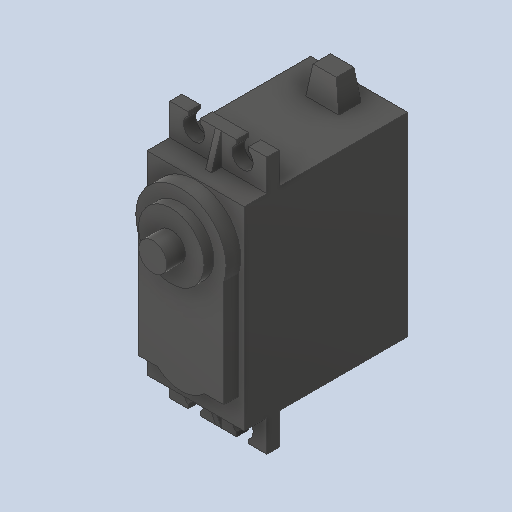
# Autodesk Inventor part: servo motor HS-7955TG
Saved by Autodesk Inventor 2022 (Build 260153000, 153)
## iProperties
Created: 2017-12-19
Part Number: servo motor HS-7955TG
Material: Generic
Document SubType Name: Modeling
Designer: s41607
Density: 1 g/cm^3
Appearance: Smooth - Dark Gray
Author: s41607
Autodesk Inventor part; units mm, degrees
ref_plane "YZ Plane" through (0, 0, 0) normal (1, 0, 0) x (0, 1, 0)
ref_plane "XZ Plane" through (0, 0, 0) normal (0, 1, 0) x (-1, 0, 0)
ref_plane "XY Plane" through (0, 0, 0) normal (0, 0, 1) x (1, 0, 0)
sketch "Sketch1" plane through (0, 0, 0) normal (0, 0, 1) x (1, 0, 0)
  line L0 (-14, 0) -> (14, 0) projected
  line L1 (0, 28) -> (0, -28) projected
  line L2 (-10, 20) -> (10, 20)
  line L3 (10, 20) -> (10, -20)
  line L4 (10, -20) -> (-10, -20)
  line L5 (-10, -20) -> (-10, 20)
  point P0 (0, 0)
  dimension "d0" = 20
  dimension "d1" = 40
  constraints: 8 end point, 2 parallel, 1 horizontal, 1 perpendicular, 2 other
  measures "d0" distance of L2.start L2.end
  measures "d1" distance of L4.end L2.start
extrude "Extrusion1" add sketch "Sketch1" along normal blind 7.2 and the other way blind 26.5
sketch "Sketch2" plane through (0, 0, 0) normal (0, 0, 1) x (1, 0, 0)
  line L0 (-14, 0) -> (14, 0) projected
  line L1 (0, 28) -> (0, -28) projected
  line L2 (-10, 20) -> (-10, -20) projected
  line L3 (10, -20) -> (10, 20) projected
  line L4 (-10, 26.5) -> (10, 26.5)
  line L5 (10, 26.5) -> (10, -26.5)
  line L6 (10, -26.5) -> (-10, -26.5)
  line L7 (-10, -26.5) -> (-10, 26.5)
  point P0 (0, 0)
  dimension "d6" = 53
  constraints: 8 end point, 2 collinear, 2 parallel, 1 horizontal, 1 perpendicular, 1 other
  measures "d6" distance of L6.end L4.start
extrude "Extrusion2" add sketch "Sketch2" along normal blind 2.5
sketch "Sketch3" plane through (0, 0, 0) normal (0, 0, 1) x (1, 0, 0)
  line L0 (0, 37.1) -> (0, -37.1) projected
  line L1 (-14, 0) -> (14, 0) projected
  line L2 (-5, 23.925) -> (5, 23.925) construction
  line L3 (5, 23.925) -> (5, -23.925) construction
  line L4 (5, -23.925) -> (-5, -23.925) construction
  line L5 (-5, -23.925) -> (-5, 23.925) construction
  point P0 (0, 0)
  dimension "d9" = 47.85
  dimension "d10" = 10
  constraints: 8 end point, 4 coincident, 2 parallel, 1 horizontal, 1 perpendicular, 2 other
  measures "d9" distance of L2.end L3.end
  measures "d10" distance of L2.start L2.end
hole "Hole1" at (5, 23.925, 0) at (-5, 23.925, 0) at (-5, -23.925, 0) at (5, -23.925, 0) direction (0, 0, 1) diameter 4.35 depth 8 tip angle 118
sketch "Sketch4" plane through (0, 0, 0) normal (0, 0, 1) x (1, 0, 0)
  line L0 (-14, 0) -> (14, 0) projected
  line L1 (0, 37.1) -> (0, -37.1) projected
  line L2 (10, 26.5) -> (-10, 26.5) projected
  line L3 (-10, -26.5) -> (10, -26.5) projected
  circle A0 centre (-5, 23.925) radius 2.175 projected
  circle A1 centre (5, 23.925) radius 2.175 projected
  circle A2 centre (-5, -23.925) radius 2.175 projected
  circle A3 centre (5, -23.925) radius 2.175 projected
  line L4 (-6.25, -23.925) -> (-3.75, -23.925)
  line L5 (-3.75, -23.925) -> (-3.75, -26.5)
  line L6 (-3.75, -26.5) -> (-6.25, -26.5)
  line L7 (-6.25, -26.5) -> (-6.25, -23.925)
  line L8 (6.25, -23.925) -> (3.75, -23.925)
  line L9 (3.75, -23.925) -> (3.75, -26.5)
  line L10 (3.75, -26.5) -> (6.25, -26.5)
  line L11 (6.25, -26.5) -> (6.25, -23.925)
  line L12 (-10, 26.5) -> (10, 26.5) projected
  line L13 (6.25, 26.5) -> (3.75, 26.5)
  line L14 (3.75, 26.5) -> (3.75, 23.925)
  line L15 (3.75, 23.925) -> (6.25, 23.925)
  line L16 (6.25, 23.925) -> (6.25, 26.5)
  line L17 (-3.75, 26.5) -> (-6.25, 26.5)
  line L18 (-6.25, 26.5) -> (-6.25, 23.925)
  line L19 (-6.25, 23.925) -> (-3.75, 23.925)
  line L20 (-3.75, 23.925) -> (-3.75, 26.5)
  point P0 (0, 0)
  dimension "d18" = 2.5
  dimension "d19" = 2.5
  dimension "d20" = 2.5
  dimension "d21" = 2.5
  constraints: 32 end point, 8 parallel, 4 coincident, 4 horizontal, 4 midpoint, 4 perpendicular, 4 point on line
  measures "d18" distance between parallel lines of L7 L5
  measures "d19" distance between parallel lines of L11 L9
  measures "d20" distance between parallel lines of L16 L14
  measures "d21" distance between parallel lines of L20 L18
extrude "Extrusion3" cut sketch "Sketch4" along normal through all contours L9 A3 L11 L3 | L3 L7 A2 L5 | L2 L16 A1 L14 | L20 A0 L18 L2 | A1 L16 L15 L14 | L20 L19 L18 A0 | A2 L7 L4 L5 | L9 L8 L11 A3 picked at (4.9114, 24.6446) picked at (-5.0886, 24.6446) picked at (-5.0886, -24.6446) picked at (4.9114, -24.6446)
sketch "Sketch5" plane through (0, 0, 0) normal (1, 0, 0) x (0, 1, 0)
  line L0 (20, 2.5) -> (26.5, 2.5) projected
  line L1 (20, 7.2) -> (20, 2.5) projected
  line L2 (26.5, 2.5) -> (20, 2.5)
  line L3 (20, 2.5) -> (20, 4.5)
  line L4 (20, 4.5) -> (26.5, 2.5)
  point P0 (0, 0)
  dimension "d24" = 2
  constraints: 6 end point, 1 horizontal, 1 point on line
  measures "d24" distance from line of L3.end L0
extrude "Extrusion4" add sketch "Sketch5" along normal mid plane 1.2
mirror "Mirror1" about plane through (0, 0, 0) normal (0, 1, 0) of "Extrusion4"
sketch "Sketch6" plane through (0, 0, 7.2) normal (0, 0, 1) x (1, 0, 0)
  line L0 (0, 37.1) -> (0, -37.1) projected
  line L1 (-14, 0) -> (14, 0) projected
  circle A0 centre (0, 10.5) radius 6.75
  line L2 (-10, -20) -> (10, -20) projected
  point P0 (0, 0)
  dimension "d27" = 30.5
  dimension "d28" = 13.5
  constraints: 1 centre point, 1 point on line
  measures "d27" distance from line of A0.centre L2
  measures "d28" diameter of A0
extrude "Extrusion5" add sketch "Sketch6" along normal blind 5
sketch "Sketch7" plane through (0, 0, 7.2) normal (0, 0, 1) x (1, 0, 0)
  circle A0 centre (0, 10.5) radius 6.75 projected
  circle A1 centre (0, 10.5) radius 9.3
  point P0 (0, 0)
  dimension "d31" = 18.6
  constraints: 1 centre point, 1 coincident
  measures "d31" diameter of A1
extrude "Extrusion6" add sketch "Sketch7" along normal blind 3
sketch "Sketch8" plane through (0, 0, 7.2) normal (0, 0, 1) x (1, 0, 0)
  line L0 (-14, 0) -> (14, 0) projected
  line L1 (0, 37.1) -> (0, -37.1) projected
  circle A0 centre (0, 10.5) radius 9.3 projected
  line L2 (-8.85, 10.5) -> (8.85, 10.5)
  line L3 (8.85, 10.5) -> (8.85, -14.4)
  line L4 (8.85, -14.4) -> (-8.85, -14.4)
  line L5 (-8.85, -14.4) -> (-8.85, 10.5)
  line L6 (10, 20) -> (-10, 20) projected
  point P0 (0, 0)
  dimension "d34" = 17.7
  dimension "d35" = 34.4
  constraints: 8 end point, 2 parallel, 1 coincident, 1 horizontal, 1 midpoint, 1 perpendicular
  measures "d34" distance of L3.end L4.end
  measures "d35" distance between parallel lines of L4 L6
extrude "Extrusion7" add sketch "Sketch8" along normal blind 3 contours L5 A0 L1 L0 | L0 L1 L4 L5 | L1 A0 L3 L0 | L0 L3 L4 L1 | L5 L2 L1 A0 | L1 L2 L3 A0 picked at (-5.9, 9.5474) picked at (5.9, 9.5474)
sketch "Sketch9" plane through (0, 0, 7.2) normal (0, 0, 1) x (1, 0, 0)
  line L0 (0, 37.1) -> (0, -37.1) projected
  line L1 (10, 20) -> (-10, 20) projected
  line L2 (-8.85, -14.4) -> (8.85, -14.4) projected
  arc A0 (-4.8, -14.4) -> (4.8, -14.4) centre (0, -9.4673) ccw
  point P0 (0, 0)
  dimension "d38" = 9.6
  dimension "d39" = 36.35
  constraints: 3 point on line, 2 point on circle, 1 centre point
  measures "d38" distance of A0.start A0.end
extrude "Extrusion8" add sketch "Sketch9" along normal blind 3
sketch "Sketch10" plane through (-10, 20, -26.5) normal (0, 1, 0) x (1, 0, 0)
  line L0 (0, 0) -> (20, 0) projected
  line L1 (10, 7.74) -> (10, -46.44) projected
  line L2 (0, -26.5) -> (20, -26.5) projected
  line L3 (20, -26.5) -> (20, 0) projected
  line L4 (0, 0) -> (20, 0) projected
  line L5 (0, 0) -> (0, -26.5) projected
  line L6 (6.6, -7.6) -> (13.4, -7.6)
  line L7 (13.4, -7.6) -> (13.4, -3)
  line L8 (13.4, -3) -> (6.6, -3)
  line L9 (6.6, -3) -> (6.6, -7.6)
  point P0 (10, -26.5)
  dimension "d42" = 3
  dimension "d43" = 4.6
  dimension "d44" = 6.8
  constraints: 8 end point, 2 parallel, 1 horizontal, 1 perpendicular, 1 other
  measures "d42" distance between parallel lines of L8 L0
  measures "d43" distance of L8.end L6.start
  measures "d44" distance of L6.start L6.end
extrude "Extrusion9" add sketch "Sketch10" along normal blind 6 contours L8 L7 L6 L1 | L1 L6 L9 L8
chamfer "Chamfer1" distance 6 distance2 1 1 edges at (3.4, 26, -21.2) measured on face at (3.4, 22, -20.4333)
chamfer "Chamfer2" distance 6 distance2 1 1 edges at (-3.4, 26, -21.2) measured on face at (-3.4, 22, -21.9667)
chamfer "Chamfer3" distance 6 distance2 0.5 1 edges at (0, 26, -18.9) measured on face at (0.8002, 22.0003, -18.9)
chamfer "Chamfer4" distance 6 distance2 0.5 1 edges at (0, 26, -23.5) measured on face at (0.8002, 22.0003, -23.5)
sketch "Sketch11" plane through (0, 10.5, 12.2) normal (0, 0, 1) x (1, 0, 0)
  circle A0 centre (0, 0) radius 6.75 projected
  circle A1 centre (0, 0) radius 2.9
  point P0 (0, -10.5)
  dimension "d59" = 5.8
  constraints: 1 centre point, 1 coincident
  measures "d59" diameter of A1
extrude "Extrusion10" add sketch "Sketch11" along normal blind 3.8 contours A1
equation "\"d19\" = d18"
equation "\"d20\" = d18"
equation "\"d21\" = d18"
body "Solid1"
